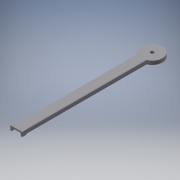
# Autodesk Inventor part: microphone2
Saved by Autodesk Inventor 2018 (Build 220112000, 112)
## iProperties
Created: 2018-02-07
Part Number: microphone2
Material: Generic
Document SubType Name: Modeling
Designer: Benedikt
Density: 1 g/cm^3
Appearance: Default
Author: Benedikt
## iProperties of the stored document microphone2_3DPrint.ipt
Created: 2018-02-07
Part Number: microphone2_3DPrint
Material: Generic
Document SubType Name: Modeling
Designer: Benedikt
Density: 1 g/cm^3
Appearance: Default
Author: Benedikt
Autodesk Inventor part; units mm, degrees
ref_plane "YZ Plane" through (0, 0, 0) normal (1, 0, 0) x (0, 1, 0)
ref_plane "XZ Plane" through (0, 0, 0) normal (0, 1, 0) x (-1, 0, 0)
ref_plane "XY Plane" through (0, 0, 0) normal (0, 0, 1) x (1, 0, 0)
sketch "Sketch1" plane through (0, 0, 0) normal (0, 1, 0) x (-1, 0, 0)
  line L0 (10.2, -1.85) -> (10.2, 0) projected
  line L1 (10.2, 0) -> (11.7, 0) projected
  line L2 (11.7, 0) -> (11.7, -4.35) projected
  line L3 (11.7, -4.35) -> (0, -4.35) projected
  line L4 (0, -4.35) -> (0, 0) projected
  line L5 (0, 0) -> (1.5, 0) projected
  line L6 (1.5, 0) -> (1.5, -1.85) projected
  arc A0 (1.5, -1.85) -> (2.5, -2.85) centre (2.5, -1.85) ccw projected
  line L7 (2.5, -2.85) -> (9.2, -2.85) projected
  arc A1 (9.2, -2.85) -> (10.2, -1.85) centre (9.2, -1.85) ccw projected
  line L8 (10.2, 1.85) -> (10.2, 0)
  line L9 (11.7, 0) -> (11.7, 4.35)
  line L10 (11.7, 4.35) -> (0, 4.35)
  line L11 (0, 4.35) -> (0, 0)
  line L12 (1.5, 0) -> (1.5, 1.85)
  arc A2 (2.5, 2.85) -> (1.5, 1.85) centre (2.5, 1.85) ccw
  line L13 (2.5, 2.85) -> (9.2, 2.85)
  arc A3 (10.2, 1.85) -> (9.2, 2.85) centre (9.2, 1.85) ccw
  constraints: 12 end point, 8 symmetric about line, 4 point on circle, 2 centre point, 2 other
extrude "Extrusion1" add sketch "Sketch1" against normal blind 4 contours L8 A3 L13 A2 L12 L5 L11 L10 L9 L1
sketch "Sketch2" plane through (0, 0, 0) normal (0, 1, 0) x (1, 0, 0)
  line L0 (-0.75, 0) -> (-0.75, 2.63) projected
  arc A0 (-0.75, 2.63) -> (-1.75, 3.63) centre (-1.75, 2.63) ccw projected
  line L1 (-1.75, 3.63) -> (-9.95, 3.63) projected
  arc A1 (-9.95, 3.63) -> (-10.95, 2.63) centre (-9.95, 2.63) ccw projected
  line L2 (-10.95, 2.63) -> (-10.95, 0) projected
  line L3 (-10.95, 0) -> (-0.75, 0) projected
  line L4 (-0.75, 0) -> (-0.75, -2.63)
  arc A2 (-1.75, -3.63) -> (-0.75, -2.63) centre (-1.75, -2.63) ccw
  line L5 (-1.75, -3.63) -> (-9.95, -3.63)
  arc A3 (-10.95, -2.63) -> (-9.95, -3.63) centre (-9.95, -2.63) ccw
  line L6 (-10.95, -2.63) -> (-10.95, 0)
  arc A4 (-7.85, 0) -> (-3.85, 0) centre (-5.85, 0) ccw
  point P0 (0, 0)
  dimension "d2" = 2
  constraints: 6 end point, 6 point on circle, 6 symmetric about line, 3 centre point, 2 point on line, 1 midpoint, 2 other
  measures "d2" radius of A4
extrude "Extrusion2" add sketch "Sketch2" along normal blind 85 contours L4 A2 L5 A3 L6 L3 A4
sketch "Sketch3" plane through (0, 85, 0) normal (0, 1, 0) x (1, 0, 0)
  point P0 (0, 0)
sketch "Sketch4" plane through (-9.95, 0, 3.63) normal (0, 0, 1) x (1, 0, 0)
  circle A0 centre (7, 90) radius 10
  line L0 (-1.75, 0) -> (9.95, 0) projected
  line L1 (9.2, 0) -> (9.2, 85) projected
  line L2 (-1, 0) -> (-1, 85) projected
  dimension "d6" = 20
  dimension "d12" = 90
  dimension "d14" = 8
  constraints: 1 centre point
  measures "d6" diameter of A0
  measures "d12" distance from line of A0.centre L0
  measures "d14" distance from line of A0.centre L2
extrude "Extrusion3" add sketch "Sketch4" against normal up to surface (3.63 mm away) contours A0
sketch "Sketch5" plane through (-9.95, 0, 3.63) normal (0, 0, 1) x (1, 0, 0)
  circle A0 centre (7, 90) radius 1.7
  circle A1 centre (7, 90) radius 10 projected
  point P0 (9.95, 0)
  point P1 (0, 82.8586)
  point P2 (8.2, 80.0723)
  dimension "d9" = 3.4
  constraints: 1 centre point, 1 concentric
  measures "d9" diameter of A0
extrude "Extrusion4" cut sketch "Sketch5" against normal blind 120 contours A0
body "Solid1"
